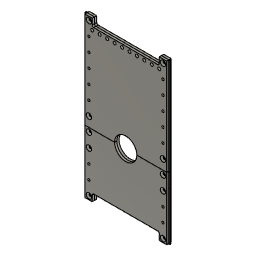
RPITower v55 (Autodesk Fusion 360 archive; units mm, degrees)
design "RPITowerSledBase"
Autodesk Fusion 360 part; units mm, degrees
sketch "Housing" plane through (0, 0, 0) normal (0, 0, 1) x (1, 0, 0)
  circle A0 centre (0, 0) radius 57.5
  line L0 (-57.5, 0) -> (57.5, 0)
  line L1 (-57.5, -1) -> (57.5, -1)
  line L2 (-57.5, 1) -> (57.5, 1)
  line L3 (-57.4217, 3) -> (-55.4217, 3)
  line L4 (-55.4217, 3) -> (-55.4217, 1)
  line L5 (-55.4217, -1) -> (-55.4217, -3)
  line L6 (-55.4217, -3) -> (-57.4217, -3)
  line L7 (57.4217, 3) -> (55.4217, 3)
  line L8 (55.4217, 3) -> (55.4217, 1)
  line L9 (55.4217, -1) -> (55.4217, -3)
  line L10 (55.4217, -3) -> (57.4217, -3)
  line L11 (-57.2217, 0.8) -> (-55.2217, 0.8)
  line L12 (-55.2217, 0.8) -> (-55.2217, 3)
  line L13 (-55.2217, 3) -> (55.2217, 3)
  line L14 (55.2217, 3) -> (55.2217, 0.8)
  line L15 (55.2217, 0.8) -> (57.2217, 0.8)
  line L16 (57.2217, 0.8) -> (57.2217, -0.8)
  line L17 (57.2217, -0.8) -> (55.2217, -0.8)
  line L18 (55.2217, -0.8) -> (55.2217, -3)
  line L19 (55.2217, -3) -> (-55.2217, -3)
  line L20 (-55.2217, -3) -> (-55.2217, -0.8)
  line L21 (-55.2217, -0.8) -> (-57.2217, -0.8)
  line L22 (-57.2217, -0.8) -> (-57.2217, 0.8)
  line L23 (-55.4217, 3) -> (-55.2217, 3)
  line L24 (-55.4217, -3) -> (-55.2217, -3)
  line L25 (55.2217, 3) -> (55.4217, 3)
  line L26 (55.2217, -3) -> (55.4217, -3)
  dimension "d12" = 115
  dimension "d14" = 1
  dimension "d15" = -1
  dimension "d16" = 2
  dimension "d17" = 2
  dimension "d18" = 2
  dimension "d19" = 2
  dimension "d20" = 2
  dimension "d21" = 2
  dimension "d22" = 2
  dimension "d23" = 2
  dimension "d24" = 0.2
  dimension "d25" = 0.2
  dimension "d26" = 0.2
  dimension "d27" = 0.2
  dimension "d30" = 0.2
  dimension "d31" = 0.2
  dimension "d32" = 0.2
  dimension "d33" = 0.2
  dimension "d121" = 2
  dimension "d122" = 2
  constraint horizontal L0
  constraint coincident A0.centre L0
  constraint coincident A0 L3.start
  constraint parallel L2 L3
  constraint coincident L2 L4.end
  constraint perpendicular L2 L4
  constraint coincident L1 L5.start
  constraint perpendicular L1 L5
  constraint coincident A0 L6.end
  constraint perpendicular L5 L6
  constraint coincident A0 L7.start
  constraint parallel L2 L7
  constraint coincident L2 L8.end
  constraint perpendicular L2 L8
  constraint coincident L1 L9.start
  constraint perpendicular L1 L9
  constraint coincident A0 L10.end
  constraint perpendicular L9 L10
  constraint parallel L0 L11
  constraint perpendicular L3 L12
  constraint perpendicular L8 L13
  constraint perpendicular L2 L14
  constraint perpendicular L8 L15
  constraint perpendicular L1 L16
  constraint perpendicular L9 L17
  constraint perpendicular L10 L18
  constraint perpendicular L5 L19
  constraint perpendicular L1 L20
  constraint perpendicular L20 L21
  constraint perpendicular L21 L22
  constraint collinear L3 L13
  constraint collinear L6 L19
  constraint coincident A0 L0.start
  constraint horizontal L2
  constraint coincident A0 L0.end
  constraint coincident A0.centre origin
  measures "d12" diameter of A0
  measures "d16" distance of L5.start L5.end
  measures "d17" distance of L3.end L4.end
  measures "d18" distance of L3.start L3.end
  measures "d19" distance of L5.end L6.end
  measures "d20" distance of L9.start L9.end
  measures "d21" distance of L7.end L8.end
  measures "d22" distance of L7.start L7.end
  measures "d23" distance of L9.end L10.end
  measures "d24" distance of L4 L12
  measures "d25" distance of L5 L20
  measures "d26" distance of L1 L21
  measures "d27" distance of L2 L11
  measures "d30" distance of L8 L14
  measures "d31" distance of L9 L18
  measures "d32" distance of L1 L17
  measures "d33" distance of L2 L15
  measures "d121" distance of L14.end L15.end
  measures "d122" distance of L11.start L11.end
extrude "Extrude9" add sketch "Housing" against normal blind 150 from surface at -25 contours L2 L12 L13 L14 | L0 L2 L11 L12 L14 L15 L16 L22 makes body 1
extrude "Extrude10" add sketch "Housing" against normal blind 130 from surface at -25 separate body contours L0 L1 L16 L17 L18 L20 L21 L22 | L1 L18 L19 L20 makes body 2
extrude "Extrude11" add 1 faces at (18.4072, 2.3333, -175) along direction (0, 0, -1) blind 64.6 separate body on bodies 1 makes body 3
extrude "Extrude12" add 1 faces at (-18.4072, -2.3333, -155) along direction (0, 0, -1) blind 84.6 separate body on bodies 2 makes body 4
sketch "SledBasics" plane through (0, -3, 0) normal (0, -1, 0) x (1, 0, 0)
  line L0 (55.2217, -25) -> (-55.2217, -25)
  line L1 (-55.2217, -25) -> (-55.2217, -155)
  line L2 (-55.2217, -155) -> (55.2217, -155)
  line L3 (55.2217, -155) -> (55.2217, -25)
  line L4 (55.2217, -155) -> (-55.2217, -155)
  line L5 (-55.2217, -155) -> (-55.2217, -239.6)
  line L6 (-55.2217, -239.6) -> (55.2217, -239.6)
  line L7 (55.2217, -239.6) -> (55.2217, -155)
  line L8 (-45.2217, -239.6) -> (45.2217, -239.6)
  line L9 (45.2217, -239.6) -> (45.2217, -229.6)
  line L10 (45.2217, -229.6) -> (-45.2217, -229.6)
  line L11 (-45.2217, -229.6) -> (-45.2217, -239.6)
  line L12 (-45.2217, -25) -> (45.2217, -25)
  line L13 (45.2217, -25) -> (45.2217, -35)
  line L14 (45.2217, -35) -> (-45.2217, -35)
  line L15 (-45.2217, -35) -> (-45.2217, -25)
  circle A0 centre (-45.2217, -39) radius 2
  circle A1 centre (-35.1661, -39) radius 2
  circle A2 centre (-25.1106, -39) radius 2
  circle A3 centre (-15.055, -39) radius 2
  circle A4 centre (-4.9995, -39) radius 2
  circle A5 centre (5.0561, -39) radius 2
  circle A6 centre (15.1116, -39) radius 2
  circle A7 centre (25.1672, -39) radius 2
  circle A8 centre (35.2228, -39) radius 2
  circle A9 centre (45.2783, -39) radius 2
  circle A10 centre (0, -155) radius 15
  circle A11 centre (-49.7217, -30) radius 1.6
  circle A12 centre (-49.7217, -30) radius 1.5
  circle A13 centre (-49.7217, -48.6364) radius 1.6
  circle A14 centre (-49.7217, -48.6364) radius 1.5
  circle A15 centre (-49.7217, -67.2727) radius 1.6
  circle A16 centre (-49.7217, -67.2727) radius 1.5
  circle A17 centre (-49.7217, -85.9091) radius 1.6
  circle A18 centre (-49.7217, -85.9091) radius 1.5
  circle A19 centre (-49.7217, -104.5455) radius 1.6
  circle A20 centre (-49.7217, -104.5455) radius 1.5
  circle A21 centre (-49.7217, -123.1818) radius 1.6
  circle A22 centre (-49.7217, -123.1818) radius 1.5
  circle A23 centre (-49.7217, -141.8182) radius 1.6
  circle A24 centre (-49.7217, -141.8182) radius 1.5
  circle A25 centre (-49.7217, -160.4545) radius 1.6
  circle A26 centre (-49.7217, -160.4545) radius 1.5
  circle A27 centre (-49.7217, -179.0909) radius 1.6
  circle A28 centre (-49.7217, -179.0909) radius 1.5
  circle A29 centre (-49.7217, -197.7273) radius 1.6
  circle A30 centre (-49.7217, -197.7273) radius 1.5
  circle A31 centre (-49.7217, -216.3636) radius 1.6
  circle A32 centre (-49.7217, -216.3636) radius 1.5
  circle A33 centre (-49.7217, -235) radius 1.6
  circle A34 centre (-49.7217, -235) radius 1.5
  circle A35 centre (50.2783, -30) radius 1.6
  circle A36 centre (50.2783, -30) radius 1.5
  circle A37 centre (50.2783, -48.6364) radius 1.6
  circle A38 centre (50.2783, -48.6364) radius 1.5
  circle A39 centre (50.2783, -67.2727) radius 1.6
  circle A40 centre (50.2783, -67.2727) radius 1.5
  circle A41 centre (50.2783, -85.9091) radius 1.6
  circle A42 centre (50.2783, -85.9091) radius 1.5
  circle A43 centre (50.2783, -104.5455) radius 1.6
  circle A44 centre (50.2783, -104.5455) radius 1.5
  circle A45 centre (50.2783, -123.1818) radius 1.6
  circle A46 centre (50.2783, -123.1818) radius 1.5
  circle A47 centre (50.2783, -141.8182) radius 1.6
  circle A48 centre (50.2783, -141.8182) radius 1.5
  circle A49 centre (50.2783, -160.4545) radius 1.6
  circle A50 centre (50.2783, -160.4545) radius 1.5
  circle A51 centre (50.2783, -179.0909) radius 1.6
  circle A52 centre (50.2783, -179.0909) radius 1.5
  circle A53 centre (50.2783, -197.7273) radius 1.6
  circle A54 centre (50.2783, -197.7273) radius 1.5
  circle A55 centre (50.2783, -216.3636) radius 1.6
  circle A56 centre (50.2783, -216.3636) radius 1.5
  circle A57 centre (50.2783, -235) radius 1.6
  circle A58 centre (50.2783, -235) radius 1.5
  dimension "d72" = 10
  dimension "d73" = 10
  dimension "d109" = 10
  dimension "d110" = 10
  dimension "d111" = 10
  dimension "d123" = 10
  dimension "d124" = 10
  dimension "d127" = 90.5
  dimension "d128" = -4
  dimension "d129" = 14
  dimension "d183" = 3.2
  dimension "d184" = 3
  dimension "d185" = 5
  dimension "d186" = 5.5
  dimension "d189" = 100
  dimension "d190" = -205
  constraint horizontal L8
  constraint vertical L9
  constraint horizontal L10
  constraint vertical L11
  constraint coincident L6 L8.start
  constraint horizontal L12
  constraint vertical L13
  constraint horizontal L14
  constraint vertical L15
  constraint coincident L0 L12.start
  constraint midpoint L4 A10.centre
  constraint concentric A11 A12
  measures "d72" distance of L8.start L10.end
  measures "d73" distance of L5.end L8.start
  measures "d109" distance of L12.start L14.end
  measures "d110" distance of L1 L15
  measures "d111" distance of L3 L13
  measures "d123" distance of L6.end L9
  measures "d124" distance of L1 A0.centre
  measures "d129" distance of L0 A0.centre
  measures "d183" diameter of A11
  measures "d184" diameter of A12
  measures "d185" distance of L0 A11.centre
  measures "d186" distance of L1 A11.centre
extrude "Extrude13" cut sketch "SledBasics" against normal blind 6 contours L0 L12 L13 L14 L15 | L2 L4 A10 | L2 L4 A10 | L6 L8 L9 L10 L11 | A0 | A1 | A2 | A3 | A4 | A5 | A6 | A7 | A8 | A9 | A12 | A14 | A16 | A18 | A20 | A22 | A24 | A26 | A28 | A30 | A32 | A34 | A36 | A38 | A40 | A42 | A44 | A46 | A48 | A50 | A52 | A54 | A56 | A58 bodies 1 2 3 4
extrude "Extrude14" cut sketch "SledBasics" against normal blind 3 contours A11 | A23 | A25 | A27 | A33 | A35 | A47 | A49 | A51 | A57 bodies 2 4
chamfer "Chamfer3" distance 2 angle 45 10 edges at (-51.2134, -3, -159.876) (-51.2134, -3, -178.5123) (48.7866, -3, -159.876) (48.7866, -3, -178.5123) (48.7866, -3, -234.4214) (-51.2134, -3, -234.4214) (-51.2134, -3, -29.4214) (48.7866, -3, -29.4214) (-51.2134, -3, -141.2396) (48.7866, -3, -141.2396) on bodies 2 4
fillet "Fillet4" radius 2 8 edges at (-45.2217, 1.5, -35) (45.2217, 1.5, -35) (-45.2217, -1.5, -35) (45.2217, -1.5, -35) (45.2217, 1.5, -229.6) (-45.2217, 1.5, -229.6) (45.2217, -1.5, -229.6) (-45.2217, -1.5, -229.6) on bodies 1 2 3 4
thread "Thread5" "ISO Metric profile 3.0 M3x0.5 6H" major diameter 3.086 minor diameter 2.529 pitch 0.5 angle 60 modelled right hand crest width 0.1368 on face at (49.594, 1, -31.3348) crest through (51.5428, 0.125, -30) on bodies 1
thread "Thread6" "ISO Metric profile 3.0 M3x0.5 6H" major diameter 3.086 minor diameter 2.529 pitch 0.5 angle 60 modelled right hand crest width 0.1368 on face at (-50.406, 1, -31.3348) crest through (-48.4572, 0.125, -30) on bodies 1
thread "Thread7" "ISO Metric profile 3.0 M3x0.5 6H" major diameter 3.086 minor diameter 2.529 pitch 0.5 angle 60 modelled right hand crest width 0.1368 on face at (-48.8461, 1, -140.6003) crest through (-48.4572, 0.125, -141.8182) on bodies 1
thread "Thread8" "ISO Metric profile 3.0 M3x0.5 6H" major diameter 3.086 minor diameter 2.529 pitch 0.5 angle 60 modelled right hand crest width 0.1368 on face at (-48.8461, 1, -159.2366) crest through (-48.4572, 0.125, -160.4545) on bodies 1
thread "Thread9" "ISO Metric profile 3.0 M3x0.5 6H" major diameter 3.086 minor diameter 2.529 pitch 0.5 angle 60 modelled right hand crest width 0.1368 on face at (-48.8461, 1, -177.873) crest through (-48.4572, 0.125, -179.0909) on bodies 3
thread "Thread10" "ISO Metric profile 3.0 M3x0.5 6H" major diameter 3.086 minor diameter 2.529 pitch 0.5 angle 60 modelled right hand crest width 0.1368 on face at (-48.8461, 1, -233.7821) crest through (-48.4572, 0.125, -235) on bodies 3
thread "Thread11" "ISO Metric profile 3.0 M3x0.5 6H" major diameter 3.086 minor diameter 2.529 pitch 0.5 angle 60 modelled right hand crest width 0.1368 on face at (51.1539, 1, -233.7821) crest through (51.5428, 0.125, -235) on bodies 3
thread "Thread12" "ISO Metric profile 3.0 M3x0.5 6H" major diameter 3.086 minor diameter 2.529 pitch 0.5 angle 60 modelled right hand crest width 0.1368 on face at (51.1539, 1, -140.6003) crest through (51.5428, 0.125, -141.8182) on bodies 1
thread "Thread13" "ISO Metric profile 3.0 M3x0.5 6H" major diameter 3.086 minor diameter 2.529 pitch 0.5 angle 60 modelled right hand crest width 0.1368 on face at (51.1539, 1, -159.2366) crest through (51.5428, 0.125, -160.4545) on bodies 1
thread "Thread14" "ISO Metric profile 3.0 M3x0.5 6H" major diameter 3.086 minor diameter 2.529 pitch 0.5 angle 60 modelled right hand crest width 0.1368 on face at (51.1539, 1, -177.873) crest through (51.5428, 0.125, -179.0909) on bodies 3
named bodies: "Sled1", "Sled2", "Sled3", "Sled4"
